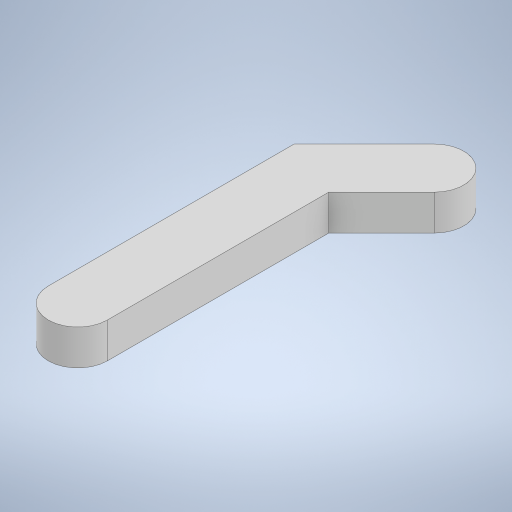
# Autodesk Inventor part: Arm 1
Saved by Autodesk Inventor 2023 (Build 270158000, 158)
## iProperties
Created: 2024-06-27
Part Number: Arm 1
Material: Generic
Document SubType Name: Modeling
Designer: Swoby
Density: 1 g/cm^3
Appearance: Default
Author: Swoby
Autodesk Inventor part; units mm, degrees
ref_plane "YZ Plane" through (0, 0, 0) normal (1, 0, 0) x (0, 1, 0)
ref_plane "XZ Plane" through (0, 0, 0) normal (0, 1, 0) x (-1, 0, 0)
ref_plane "XY Plane" through (0, 0, 0) normal (0, 0, 1) x (1, 0, 0)
sketch "Sketch1" plane through (0, 0, 0) normal (0, 1, 0) x (-1, 0, 0)
  circle A0 centre (0, 0) radius 25
  line L0 (25, 0) -> (25, -208.3553)
  line L1 (25, -208.3553) -> (-34.3223, -267.6777)
  line L2 (-25, 0) -> (-25, -187.6447)
  line L3 (-25, -187.6447) -> (-69.6777, -232.3223)
  circle A1 centre (-52, -250) radius 25
  dimension "d0" = 50
  dimension "d1" = 50
  dimension "d2" = 250
  dimension "d3" = 27
  dimension "d4" = 135
  constraints: 8 end point, 4 point on circle, 4 tangent, 2 centre point, 2 parallel, 1 coincident, 1 vertical
  measures "d0" diameter of A0
  measures "d1" diameter of A1
  measures "d2" vertical distance of point (0, 0) A1.centre
  measures "d3" distance from line of L2 A1.centre
  measures "d4" angle of L1 L0
extrude "Extrusion1" add sketch "Sketch1" along normal blind 30
body "Solid1"
